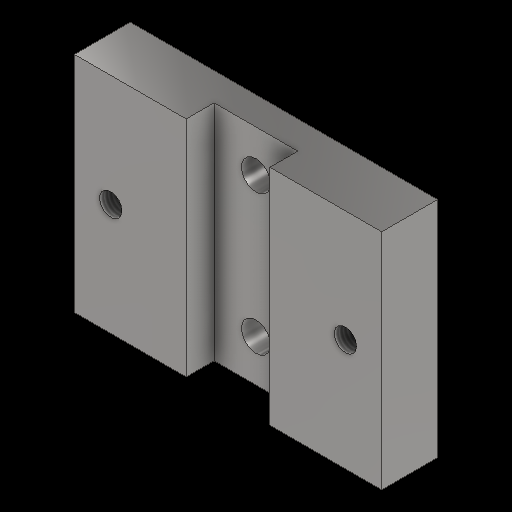
# Autodesk Inventor part: Leadscrew Bearing Bracket
Saved by Autodesk Inventor 2026.1 (Build 301233000, 233)
## iProperties
Created: 2024-12-30
Part Number: Leadscrew Bearing Bracket
Material: Stainless Steel
Document SubType Name: Modeling
Designer: drago
Density: 8 g/cm^3
Appearance: Semi-Polished
Mass: 148.29 g
Surface Area: 68.2948 cm^2
Volume: 18.5363 cm^3
Author: drago
Autodesk Inventor part; units mm, degrees
ref_plane "YZ Plane" through (0, 0, 0) normal (1, 0, 0) x (0, 1, 0)
ref_plane "XZ Plane" through (0, 0, 0) normal (0, 1, 0) x (-1, 0, 0)
ref_plane "XY Plane" through (0, 0, 0) normal (0, 0, 1) x (1, 0, 0)
sketch "Sketch2" plane through (0, 0, 0) normal (0, 0, 1) x (1, 0, 0)
  line L0 (0, 0) -> (55, 0)
  line L1 (55, 0) -> (55, 40)
  line L2 (55, 40) -> (0, 40)
  line L3 (0, 40) -> (0, 0)
  line L4 (35, 40) -> (35, 0)
  line L5 (20, 40) -> (20, 0)
  line L6 (0, 20) -> (55, 20) construction
  line L7 (27.5, 0) -> (27.5, 40) construction
  circle A0 centre (6.5, 20) radius 2
  circle A1 centre (48.5, 20) radius 2
  circle A2 centre (27.5, 7.5) radius 2.6
  circle A3 centre (27.5, 32.5) radius 2.6
  point P0 (27.5, 7.5)
  point P1 (6.5, 20)
  point P2 (27.5, 32.5)
  dimension "d19" = 55
  dimension "d20" = 40
  dimension "d21" = 20
  dimension "d23" = 6.5
  dimension "d24" = 7.5
  dimension "d25" = 4
  dimension "d26" = 5.2
  constraints: 16 end point, 8 point on line, 5 coincident, 4 centre point, 4 midpoint, 3 perpendicular, 2 equal radius, 2 parallel, 2 symmetric about line, 1 horizontal, 4 other
  measures "d19" distance of L2.end L1.end
  measures "d20" distance of L1.end L0.end
  measures "d21" distance between parallel lines of L5 L3
  measures "d23" distance from line of L3 point (6.5, 20)
  measures "d24" distance from line of L2 point (27.5, 32.5)
  measures "d25" diameter of A0
  measures "d26" diameter of A2
extrude "Extrusion1" add sketch "Sketch2" against normal blind 10 contours L3 L2 L5 L0 | L5 L2 L4 L0 | L4 L2 L1 L0 | A0 | A1 | A2 | A3
extrude "Extrusion2" cut sketch "Sketch2" against normal blind 5 contours L5 L2 L4 L0
hole "Hole1" at (6.5, 20, 0) at (48.5, 20, 0) direction (0, 0, -1) diameter 4 end through all
hole "Hole2" at (27.5, 7.5, 0) at (27.5, 32.5, 0) direction (0, 0, -1) diameter 5.2 end through all
thread "Thread3" size "M4x0.7" class "6H" standard "ISO Metric profile" full length
thread "Thread4" size "M4x0.7" class "6H" standard "ISO Metric profile" full length
body "Solid3"
